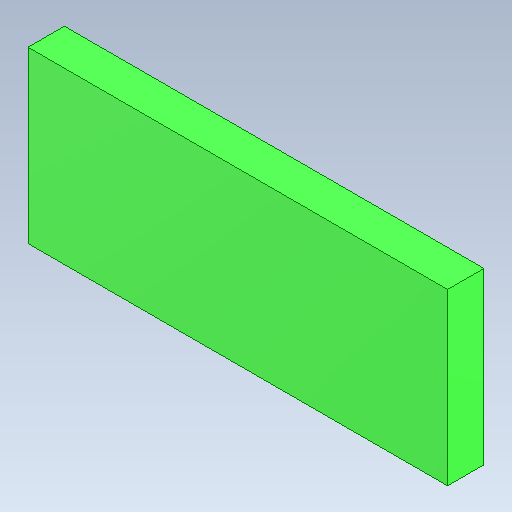
# Autodesk Inventor part: 16MHZ
Saved by Autodesk Inventor 2020 (Build 240168000, 168)
## iProperties
Created: 2019-05-24
Part Number: 16MHZ
Material: Generic
Document SubType Name: Modeling
Designer: psrob
Density: 1 g/cm^3
Appearance: HC49US, 16MHZ
Author: psrob
Autodesk Inventor part; units mm, degrees
ref_plane "YZ Plane" through (0, 0, 0) normal (1, 0, 0) x (0, 1, 0)
ref_plane "XZ Plane" through (0, 0, 0) normal (0, 1, 0) x (-1, 0, 0)
ref_plane "XY Plane" through (0, 0, 0) normal (0, 0, 1) x (1, 0, 0)
sketch "HC49US, 16MHZ_63" plane through (0, 0, 0) normal (0, 0, 1) x (1, 0, 0)
  line L0 (-5.8166, 2.286) -> (5.715, 2.286)
  line L1 (5.715, 2.286) -> (5.715, -2.3876)
  line L2 (5.715, -2.3876) -> (-5.8166, -2.3876)
  line L3 (-5.8166, -2.3876) -> (-5.8166, 2.286)
  constraints: 8 end point
extrude "Extrusion1" add sketch "HC49US, 16MHZ_63" along normal blind 1
body "Solid1"
